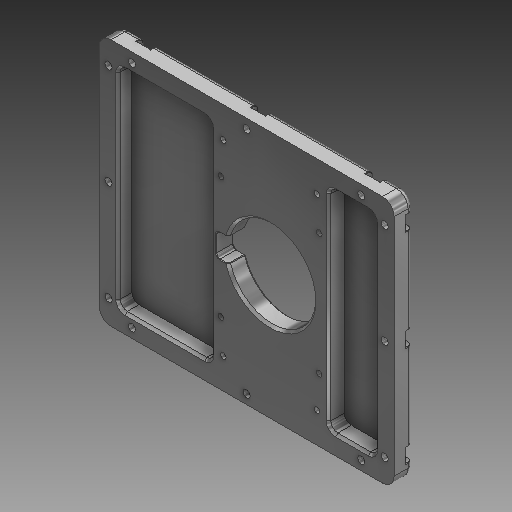
# Autodesk Inventor part: Top motor plate
Saved by Autodesk Inventor 2019 (Build 230136000, 136)
## iProperties
Created: 2018-05-03
Part Number: Top motor plate
Material: Aluminum 6061
Document SubType Name: Modeling
Designer: SimonD
Density: 2.7 g/cm^3
Appearance: Aluminum - Polished
Author: SimonD
Autodesk Inventor part; units mm, degrees
ref_plane "YZ Plane" through (0, 0, 0) normal (1, 0, 0) x (0, 1, 0)
ref_plane "XZ Plane" through (0, 0, 0) normal (0, 1, 0) x (-1, 0, 0)
ref_plane "XY Plane" through (0, 0, 0) normal (0, 0, 1) x (1, 0, 0)
sketch "Sketch1" plane through (0, 0, 0) normal (0, 0, 1) x (1, 0, 0)
  line L0 (-53, 53) -> (53, 53)
  line L1 (53, 53) -> (53, -53)
  line L2 (53, -53) -> (-53, -53)
  line L3 (-53, -53) -> (-53, 53)
  line L4 (-53, 53) -> (53, -53) construction
  line L5 (53, 53) -> (-53, -53) construction
  point P0 (0, 0)
  dimension "d0" = 106
  dimension "d1" = 106
  constraints: 12 end point, 2 midpoint, 2 parallel, 1 horizontal, 1 perpendicular
  measures "d0" distance of L1.end L2.end
  measures "d1" distance between parallel lines of L2 L0
extrude "Extrusion1" add sketch "Sketch1" along normal blind 8
sketch "Sketch2" plane through (0, 0, 8) normal (0, 0, 1) x (1, 0, 0)
  circle A0 centre (0, 0) radius 18.6
  dimension "d4" = 37.2
  constraints: 1 centre point, 1 coincident
  measures "d4" diameter of A0
extrude "Extrusion2" cut sketch "Sketch2" against normal blind 8
thicken "Thicken1" operation add thickness 20 both sides no extend neighbours yes toward (-1, 0, 0) faces at (-53, -17.6667, 5.3333)
fillet "Fillet4" radius 5 4 edges at (53, -53, 4) (53, 53, 4) (-73, 53, 4) (-73, -53, 4)
sketch "Sketch8" plane through (0, 0, 0) normal (0, 0, -1) x (-1, 0, 0)
  line L0 (73, 48) -> (73, -48) projected
  line L1 (68, -53) -> (-48, -53) projected
  line L2 (-53, -48) -> (-53, 48) projected
  line L3 (68, 53) -> (-48, 53) projected
  point P0 (0, 0)
  point P1 (-39, 49)
  point P2 (-49, 0)
  point P3 (-39, -49)
  point P4 (10, -49)
  point P5 (10, 49)
  point P6 (-49, 43)
  point P7 (-49, -43)
  point P8 (59, 49)
  point P9 (69, 0)
  point P10 (69, -43)
  point P11 (59, -49)
  point P12 (69, 43)
  dimension "d215" = 63
  dimension "d216" = 14
  dimension "d217" = 4
  dimension "d218" = 4
  dimension "d219" = 14
  dimension "d220" = 4
  dimension "d221" = 4
  dimension "d222" = 63
  dimension "d223" = 14
  dimension "d224" = 10
  dimension "d225" = 4
  dimension "d226" = 10
  dimension "d227" = 4
  dimension "d228" = 14
  dimension "d229" = 10
  dimension "d230" = 10
  dimension "d246" = 4
  dimension "d247" = 4
  measures "d215" distance from line of point (10, -49) L2
  measures "d216" distance from line of point (59, -49) L0
  measures "d217" distance from line of point (59, -49) L1
  measures "d218" distance from line of point (69, -43) L0
  measures "d219" distance from line of point (59, 49) L0
  measures "d220" distance from line of point (59, 49) L3
  measures "d221" distance from line of point (10, 49) L3
  measures "d222" distance from line of point (10, 49) L0
  measures "d223" distance from line of point (-39, 49) L2
  measures "d224" distance from line of point (-49, 43) L3
  measures "d225" distance from line of point (-49, 43) L2
  measures "d226" distance from line of point (-49, -43) L1
  measures "d227" distance from line of point (-39, -49) L1
  measures "d228" distance from line of point (-39, -49) L2
  measures "d229" distance from line of point (69, -43) L1
  measures "d230" distance from line of point (69, 43) L3
  measures "d246" distance from line of point (69, 43) L0
  measures "d247" distance from line of point (69, 0) L0
hole "Hole4" at (39, 49, 0) at (49, 0, 0) at (39, -49, 0) at (-10, -49, 0) at (-10, 49, 0) at (49, 43, 0) at (49, -43, 0) at (-59, 49, 0) at (-69, 43, 0) at (-69, 0, 0) at (-69, -43, 0) at (-59, -49, 0) direction (0, 0, 1) diameter 3.1 end through all
sketch "Sketch9" plane through (0, 0, 0) normal (0, 0, -1) x (-1, 0, 0)
  circle A0 centre (10, 49) radius 1.55 projected
  arc A1 (7, 49) -> (13, 49) centre (10, 49) ccw
  circle A2 centre (10, -49) radius 1.55 projected
  arc A3 (13, -49) -> (7, -49) centre (10, -49) ccw
  circle A4 centre (-39, -49) radius 1.55 projected
  line L0 (7, -49) -> (7, -53)
  line L1 (-48, -53) -> (68, -53) projected
  line L2 (13, -53) -> (13, -49)
  line L3 (7, 49) -> (7, 53)
  line L4 (7, 53) -> (13, 53)
  line L5 (13, 49) -> (13, 53)
  arc A5 (-49, -3) -> (-49, 3) centre (-49, 0) ccw
  line L6 (-49, 3) -> (-53, 3)
  line L7 (-53, -3) -> (-49, -3)
  arc A6 (-36, -49) -> (-42, -49) centre (-39, -49) ccw
  line L8 (-42, -49) -> (-42, -53)
  line L9 (-36, -49) -> (-36, -53)
  line L10 (-53, 3) -> (-53, -3)
  line L11 (-53, 48) -> (-53, -48) projected
  line L12 (-53, 46) -> (-46, 46)
  line L13 (-46, 46) -> (-46, 40)
  line L14 (-46, 40) -> (-53, 40)
  line L15 (-53, 40) -> (-53, 46)
  line L16 (-53, -40) -> (-46, -40)
  line L17 (-46, -40) -> (-46, -46)
  line L18 (-46, -46) -> (-53, -46)
  line L19 (-53, -46) -> (-53, -40)
  line L20 (68, -53) -> (-48, -53) projected
  line L21 (56, -53) -> (62, -53)
  line L22 (62, -53) -> (62, -46)
  line L23 (62, -46) -> (56, -46)
  line L24 (56, -46) -> (56, -53)
  line L25 (74, -3) -> (66, -3)
  line L26 (66, -3) -> (66, 3)
  line L27 (66, 3) -> (74, 3)
  line L28 (74, 3) -> (74, -3)
  line L29 (56, 53) -> (62, 53)
  line L30 (62, 53) -> (62, 46)
  line L31 (62, 46) -> (56, 46)
  line L32 (56, 46) -> (56, 53)
  line L33 (73, -40) -> (66, -40)
  line L34 (66, -40) -> (66, -46)
  line L35 (66, -46) -> (73, -46)
  line L36 (73, -46) -> (73, -40)
  circle A7 centre (-49, 43) radius 1.55 projected
  circle A8 centre (-49, -43) radius 1.55 projected
  circle A9 centre (59, -49) radius 1.55 projected
  circle A10 centre (59, 49) radius 1.55 projected
  circle A11 centre (69, 43) radius 1.55 projected
  circle A12 centre (69, 0) radius 1.55 projected
  circle A13 centre (69, -43) radius 1.55 projected
  line L37 (73, 48) -> (73, -48) projected
  line L38 (66, 46) -> (73, 46)
  line L39 (73, 46) -> (73, 40)
  line L40 (73, 40) -> (66, 40)
  line L41 (66, 40) -> (66, 46)
  line L42 (-42, 54.45) -> (-36, 54.45)
  line L43 (-36, 54.45) -> (-36, 46)
  line L44 (-36, 46) -> (-42, 46)
  line L45 (-42, 46) -> (-42, 54.45)
  circle A14 centre (-39, 49) radius 1.55 projected
  point P0 (0, 0)
  point P1 (-35, 49)
  point P2 (73, 3)
  point P3 (76, -53)
  point P4 (82, -53)
  dimension "d92" = 6
  dimension "d96" = 6
  dimension "d112" = 6
  dimension "d232" = 3
  dimension "d233" = 3
  dimension "d234" = 3
  dimension "d235" = 3
  dimension "d236" = 3
  dimension "d237" = 3
  dimension "d238" = 3
  dimension "d239" = 3
  dimension "d240" = 3
  dimension "d241" = 3
  dimension "d242" = 3
  dimension "d243" = 3
  dimension "d244" = 3
  dimension "d245" = 3
  dimension "d251" = 3
  dimension "d252" = 3
  dimension "d253" = 3
  constraints: 84 end point, 18 point on line, 17 parallel, 12 coincident, 12 perpendicular, 9 horizontal, 8 point on circle, 4 centre point, 4 tangent
  measures "d92" diameter of A1
  measures "d96" diameter of A3
  measures "d112" diameter of A6
  measures "d232" distance from line of L13 point (-49, 43)
  measures "d233" distance from line of L12 point (-49, 43)
  measures "d234" distance from line of L14 A7.centre
  measures "d235" distance from line of L16 point (-49, -43)
  measures "d236" distance from line of L18 A8.centre
  measures "d237" distance from line of L24 point (59, -49)
  measures "d238" distance from line of L22 A9.centre
  measures "d239" distance from line of L34 point (69, -43)
  measures "d240" distance from line of L26 point (69, 0)
  measures "d241" distance from line of L25 point (69, 0)
  measures "d242" distance from line of L27 point (69, 0)
  measures "d243" distance from line of L41 point (69, 43)
  measures "d244" distance from line of L38 point (69, 43)
  measures "d245" distance from line of L40 A11.centre
  measures "d251" distance from line of L44 point (-39, 49)
  measures "d252" distance from line of L45 point (-39, 49)
  measures "d253" distance from line of L43 point (-39, 49)
sketch "Sketch13" plane through (0, 0, 8) normal (0, 0, 1) x (1, 0, 0)
  line L0 (-73, 48) -> (-73, -48) projected
  line L1 (53, -48) -> (53, 48) projected
  point P0 (0, 0)
  point P1 (-69, 25)
  point P2 (-69, -25)
  point P3 (49, -25)
  point P4 (49, 25)
  dimension "d160" = 25
  dimension "d161" = 4
  dimension "d162" = 4
  dimension "d163" = 25
  dimension "d164" = 25
  dimension "d165" = 4
  dimension "d166" = 25
  dimension "d167" = 4
  measures "d160" vertical distance of point (-69, 25) point (0, 0)
  measures "d161" distance from line of point (-69, 25) L0
  measures "d162" distance from line of point (-69, -25) L0
  measures "d163" vertical distance of point (-69, -25) point (0, 0)
  measures "d164" vertical distance of point (49, 25) point (0, 0)
  measures "d165" distance from line of point (49, 25) L1
  measures "d166" vertical distance of point (49, -25) point (0, 0)
  measures "d167" distance from line of point (49, -25) L1
hole "Hole7" [suppressed]
sketch "Sketch16" plane through (0, 0, 8) normal (0, 0, 1) x (1, 0, 0)
  line L0 (-25, -45) -> (-65, -45)
  line L1 (-65, -45) -> (-65, 45)
  line L2 (-65, 45) -> (-25, 45)
  line L3 (-25, 45) -> (-25, -45)
  line L4 (-73, 48) -> (-73, -48) projected
  point P0 (0, 0)
  dimension "d186" = 25
  dimension "d187" = 8
  dimension "d188" = 45
  dimension "d189" = 45
  constraints: 8 end point, 2 parallel, 1 horizontal, 1 perpendicular
  measures "d186" distance from line of L3 point (0, 0)
  measures "d187" distance between parallel lines of L4 L1
  measures "d188" distance from line of L0 point (0, 0)
  measures "d189" distance from line of L2 point (0, 0)
extrude "Extrusion13" cut sketch "Sketch16" against normal blind 6
fillet "Fillet9" radius 3 4 edges at (-25, -45, 5) (-65, -45, 5) (-25, 45, 5) (-65, 45, 5)
sketch "Sketch17" plane through (0, 0, 8) normal (0, 0, 1) x (1, 0, 0)
  line L0 (45, -45) -> (25, -45)
  line L1 (25, -45) -> (25, 45)
  line L2 (25, 45) -> (45, 45)
  line L3 (45, 45) -> (45, -45)
  line L4 (53, -48) -> (53, 48) projected
  point P0 (0, 0)
  dimension "d193" = 45
  dimension "d194" = 45
  dimension "d195" = 8
  dimension "d196" = 20
  constraints: 8 end point, 2 parallel, 1 horizontal, 1 perpendicular
  measures "d193" distance from line of L0 point (0, 0)
  measures "d194" distance from line of L2 point (0, 0)
  measures "d195" distance between parallel lines of L4 L3
  measures "d196" distance between parallel lines of L1 L3
extrude "Extrusion14" cut sketch "Sketch17" against normal blind 6.75
fillet "Fillet10" radius 3 4 edges at (25, -45, 4.625) (45, -45, 4.625) (45, 45, 4.625) (25, 45, 4.625)
sketch "Sketch18" plane through (0, 0, 0) normal (0, 0, -1) x (-1, 0, 0)
  point P0 (0, 0)
  point P1 (-20, 40)
  point P2 (20, 40)
  point P3 (20, -40)
  point P4 (-20, -40)
  dimension "d200" = 40
  dimension "d201" = 20
  dimension "d202" = 20
  dimension "d203" = 40
  dimension "d204" = 40
  dimension "d205" = 20
  dimension "d206" = 20
  dimension "d207" = 40
  measures "d200" vertical distance of point (-20, 40) point (0, 0)
  measures "d201" horizontal distance of point (-20, 40) point (0, 0)
  measures "d202" horizontal distance of point (20, 40) point (0, 0)
  measures "d203" vertical distance of point (20, 40) point (0, 0)
  measures "d204" vertical distance of point (-20, -40) point (0, 0)
  measures "d205" horizontal distance of point (0, 0) point (-20, -40)
  measures "d206" horizontal distance of point (20, -40) point (0, 0)
  measures "d207" vertical distance of point (20, -40) point (0, 0)
hole "Hole8" at (20, 40, 0) at (-20, 40, 0) at (-20, -40, 0) at (20, -40, 0) direction (0, 0, 1) diameter 2.459 end through all thread size "M3x0.5" class "6H" standard "ISO Metric profile"
extrude "Extrusion16" cut sketch "Sketch9" against normal blind 3.2
fillet "Fillet12" radius 3 16 edges at (-62, -46, 1.6) (-56, -46, 1.6) (-66, -46, 1.6) (-66, -40, 1.6) (-66, -3, 1.6) (-66, 3, 1.6) (-66, 40, 1.6) (-66, 46, 1.6) (-62, 46, 1.6) (-56, 46, 1.6) (42, 46, 1.6) (36, 46, 1.6) (46, 40, 1.6) (46, 46, 1.6) (46, -46, 1.6) (46, -40, 1.6)
chamfer "Chamfer2" distance 1 angle 45 18 edges at (-18.6, 0, 8) (25, 0, 8) (25.8787, 44.1213, 8) (35, 45, 8) (44.1213, 44.1213, 8) (45, 0, 8) (44.1213, -44.1213, 8) (35, -45, 8) (25.8787, -44.1213, 8) (-45, 45, 8) (-25.8787, 44.1213, 8) (-25, 0, 8) (-25.8787, -44.1213, 8) (-45, -45, 8) (-64.1213, -44.1213, 8) (-65, 0, 8) (-64.1213, 44.1213, 8) (-18.6, 0, 0)
sketch "Sketch19" plane through (0, 0, 8) normal (0, 0, 1) x (1, 0, 0)
  point P0 (0, 0)
  point P1 (21, -26)
  point P2 (-21, -26)
  point P3 (-21, 26)
  point P4 (21, 26)
  dimension "d260" = 21
  dimension "d261" = 21
  dimension "d262" = 21
  dimension "d263" = 21
  dimension "d264" = 26
  dimension "d265" = 26
  dimension "d266" = 26
  dimension "d267" = 26
  measures "d260" horizontal distance of point (21, -26) point (0, 0)
  measures "d261" horizontal distance of point (-21, -26) point (0, 0)
  measures "d262" horizontal distance of point (21, 26) point (0, 0)
  measures "d263" horizontal distance of point (-21, 26) point (0, 0)
  measures "d264" vertical distance of point (21, -26) point (0, 0)
  measures "d265" vertical distance of point (-21, -26) point (0, 0)
  measures "d266" vertical distance of point (21, 26) point (0, 0)
  measures "d267" vertical distance of point (-21, 26) point (0, 0)
hole "Hole9" at (21, -26, 8) at (-21, -26, 8) at (-21, 26, 8) at (21, 26, 8) direction (0, 0, -1) diameter 2.459 depth 6 thread size "M3x0.5" class "6H" standard "ISO Metric profile"
sketch "Sketch20" plane through (0, 0, 8) normal (0, 0, 1) x (1, 0, 0)
  point P0 (0, 0)
  point P1 (13, -26)
  point P2 (-13, 26)
hole "Hole10" [suppressed]
fillet "Fillet14" radius 2 20 edges at (-73, 21.5, 0) (-73, -21.5, 0) (-65, -53, 0) (-73, -47, 0) (-71.5355, -51.5355, 0) (-34.5, -53, 0) (14.5, -53, 0) (53, -47, 0) (45, -53, 0) (51.5355, -51.5355, 0) (53, -21.5, 0) (53, 21.5, 0) (45, 53, 0) (53, 47, 0) (51.5355, 51.5355, 0) (14.5, 53, 0) (-34.5, 53, 0) (-71.5355, 51.5355, 0) (-73, 47, 0) (-65, 53, 0)
sketch "Sketch21" plane through (0, 0, 0) normal (0, 0, -1) x (-1, 0, 0)
  line L0 (16.5403, 5) -> (23.0403, 5)
  line L1 (23.0403, 5) -> (23.0403, -5)
  line L2 (23.0403, -5) -> (16.5403, -5)
  line L3 (16.5403, -5) -> (16.5403, 5)
  point P0 (0, 0)
  dimension "d286" = 6.5
  dimension "d288" = 5
  dimension "d289" = 5
  constraints: 8 end point, 2 parallel, 1 horizontal, 1 perpendicular
  measures "d286" distance between parallel lines of L1 L3
  measures "d288" distance from line of L2 point (0, 0)
  measures "d289" distance from line of L0 point (0, 0)
extrude "Extrusion17" cut sketch "Sketch21" against normal blind 10
fillet "Fillet15" radius 1.5 2 edges at (-23.0403, -5, 4) (-23.0403, 5, 4)
chamfer "Chamfer3" distance 1 angle 45 5 edges at (-20.2459, 5, 0) (-22.601, 4.5607, 0) (-23.0403, 0, 0) (-22.601, -4.5607, 0) (-20.2459, -5, 0)
chamfer "Chamfer4" distance 0.25 angle 45 100 edges at (-56, -50, 0) (-61.1213, -46.8787, 0) (-59, -46, 0) (-56.8787, -46.8787, 0) (-62, -50, 0) (-62, -52.4142, 0.5858) (-62, -53, 2.6) (-56, -52.4142, 0.5858) (-56, -53, 2.6) (-66.8787, -40.8787, 0) (-66, -43, 0) (-66.8787, -45.1213, 0) (-70, -46, 0) (-72.4142, -46, 0.5858) (-73, -46, 2.6) (-70, -40, 0) (-72.4142, -40, 0.5858) (-73, -40, 2.6) (-66.8787, 2.1213, 0) (-66, 0, 0) (-66.8787, -2.1213, 0) (-70, -3, 0) (-72.4142, -3, 0.5858) (-73, -3, 2.6) (-70, 3, 0) (-72.4142, 3, 0.5858) (-73, 3, 2.6) (-72.4142, 40, 0.5858) (-70, 40, 0) (-66.8787, 45.1213, 0) (-66, 43, 0) (-66.8787, 40.8787, 0) (-70, 46, 0) (-72.4142, 46, 0.5858) (-73, 46, 2.6) (-73, 40, 2.6) (-56.8787, 46.8787, 0) (-59, 46, 0) (-61.1213, 46.8787, 0) (-62, 49.9999, 0) (-62, 52.4142, 0.5858) (-62, 53, 2.6) (-56, 49.9999, 0) (-56, 52.4142, 0.5858) (-56, 53, 2.6) (-10, 46, 0) (-7, 50, 0) (-7, 52.4142, 0.5858) (-7, 53, 2.6) (-13, 50, 0) (-13, 52.4142, 0.5858) (-13, 53, 2.6) (41.1213, 46.8787, 0) (39, 46, 0) (36.8787, 46.8787, 0) (36, 49.9999, 0) (36, 52.4142, 0.5858) (36, 53, 2.6) (42, 49.9999, 0) (42, 52.4142, 0.5858) (42, 53, 2.6) (46.8787, 40.8787, 0) (46, 43, 0) (46.8787, 45.1213, 0) (49.9999, 46, 0) (52.4142, 46, 0.5858) (53, 46, 2.6) (49.9999, 40, 0) (52.4142, 40, 0.5858) (53, 40, 2.6) (46, 0, 0) (50, -3, 0) (52.4142, -3, 0.5858) (53, -3, 2.6) (50, 3, 0) (52.4142, 3, 0.5858) (53, 3, 2.6) (46.8787, -45.1213, 0) (46, -43, 0) (46.8787, -40.8787, 0) (49.9999, -40, 0) (52.4142, -40, 0.5858) (53, -40, 2.6) (49.9999, -46, 0) (52.4142, -46, 0.5858) (53, -46, 2.6) (39, -46, 0) (36, -50, 0) (36, -52.4142, 0.5858) (36, -53, 2.6) (42, -50, 0) (42, -52.4142, 0.5858) (42, -53, 2.6) (-10, -46, 0) (-13, -50, 0) (-13, -52.4142, 0.5858) (-13, -53, 2.6) (-7, -50, 0) (-7, -52.4142, 0.5858) (-7, -53, 2.6)
chamfer "Chamfer5" distance 0.2 angle 45 2 edges at (-17.9154, 5, 4) (-17.9154, -5, 4)
chamfer "Chamfer6" distance 0.25 angle 45 7 edges at (-20.2459, -5, 8) (-22.601, -4.5607, 8) (-23.0403, 0, 8) (-22.601, 4.5607, 8) (-20.2459, 5, 8) (-18.529, 5, 7.5918) (-18.529, -5, 7.5918)
body "Solid1"
